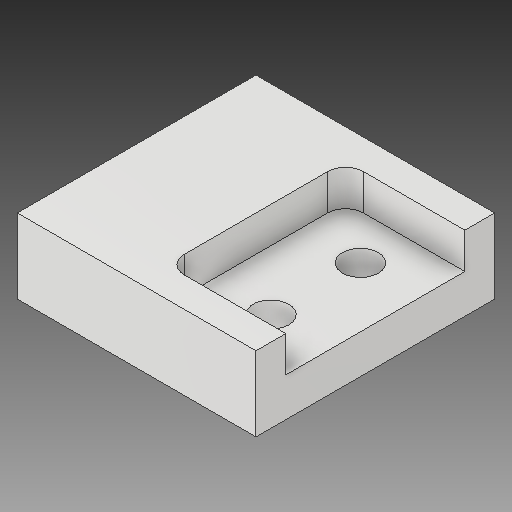
# Autodesk Inventor part: pillar_block
Saved by Autodesk Inventor 2018 (Build 220112000, 112)
## iProperties
Created: 2017-02-15
Part Number: pillar_block
Material: Aluminum 2014-T4
Document SubType Name: Modeling
Designer: steve
Density: 2.8 g/cm^3
Appearance: Satin
Mass: 5.00958 g
Surface Area: 15.2482 cm^2
Volume: 1.78914 cm^3
stock_6_width: 6,250 mm
pillar_block_length: 20,000 mm
pillar_block_width: 20,000 mm
pillar_width: 15,000 mm
stock_3_width: 3,000 mm
pillar_length: 80,000 mm
pillar_plate_length: 60,000 mm
Author: steve
Autodesk Inventor part; units mm, degrees
ref_plane "YZ Plane" through (0, 0, 0) normal (1, 0, 0) x (0, 1, 0)
ref_plane "XZ Plane" through (0, 0, 0) normal (0, 1, 0) x (-1, 0, 0)
ref_plane "XY Plane" through (0, 0, 0) normal (0, 0, 1) x (1, 0, 0)
sketch "Sketch1" plane through (0, 0, 0) normal (0, 1, 0) x (-1, 0, 0)
  line L0 (-10, -10) -> (10, -10)
  line L1 (10, -10) -> (10, 10)
  line L2 (10, 10) -> (-10, 10)
  line L3 (-10, 10) -> (-10, -10)
  line L4 (-10, -10) -> (10, 10) construction
  line L5 (10, -10) -> (-10, 10) construction
  point P0 (0, 0)
  dimension "d0" = 20
  dimension "d1" = 20
  constraints: 12 end point, 2 midpoint, 2 parallel, 1 horizontal, 1 perpendicular
  measures "d0" distance of L0.end L1.end
  measures "d1" distance of L0.start L0.end
extrude "Extrusion1" add sketch "Sketch1" along normal blind 6.25
sketch "Sketch2" plane through (0, 6.25, 0) normal (0, 1, 0) x (1, 0, 0)
  line L0 (10, -7.5) -> (0, -7.5)
  line L1 (0, -7.5) -> (0, 7.5)
  line L2 (0, 7.5) -> (10, 7.5)
  line L3 (10, 7.5) -> (10, -7.5)
  line L4 (10, -10) -> (10, 10) projected
  line L5 (0, 0) -> (15, 0) construction
  line L6 (-15, 0) -> (20, 0) construction
  line L7 (-10, 10) -> (-10, -10) construction
  point P0 (0, 0)
  dimension "d4" = 15
  dimension "d5" = 10
  constraints: 10 end point, 2 collinear, 2 parallel, 1 horizontal, 1 midpoint, 1 perpendicular
  measures "d4" distance of L0.end L1.end
  measures "d5" distance between parallel lines of L7 L1
extrude "Extrusion2" cut sketch "Sketch2" against normal blind 3
sketch "Sketch3" plane through (0, 3.25, 0) normal (0, 1, 0) x (1, 0, 0)
  line L0 (-14, 0) -> (14, 0) construction
  line L1 (10, -7.5) -> (0, -7.5) construction
  line L2 (10, -7.5) -> (0, -7.5) construction
  line L3 (5, -7.5) -> (5, 18.284) construction
  point P0 (0, 0)
  point P1 (5, -3.75)
  point P2 (5, 3.75)
  dimension "d8" = 7.5
  dimension "d26" = 3.75
  constraints: 2 end point, 2 point on line, 1 midpoint, 1 vertical
  measures "d8" distance of point (5, 3.75) point (5, -3.75)
  measures "d26" distance from line of L0 point (5, 3.75)
hole "Hole1" at (5, 3.25, 3.75) at (5, 3.25, -3.75) direction (0, -1, 0) diameter 3 end through all
sketch "Sketch4" plane through (-10, 0, -10) normal (-1, 0, 0) x (0, 0, 1)
  line L0 (0, 0) -> (20, 0) construction
  line L1 (20, 0) -> (20, 6.25) construction
  line L2 (0, 6.25) -> (20, 6.25) construction
  line L3 (0, 0) -> (0, 6.25) construction
  line L4 (20, 3.125) -> (0, 3.125) construction
  line L5 (10, 0) -> (10, 6.25) construction
  point P0 (16, 3.125)
  point P1 (4, 3.125)
  dimension "d17" = 6
  dimension "d18" = 6
  constraints: 4 end point, 3 midpoint, 2 point on line
  measures "d17" distance from line of L5 point (16, 3.125)
  measures "d18" distance from line of point (4, 3.125) L5
hole "Hole2" at (-10, 3.125, 6) at (-10, 3.125, -6) direction (1, 0, 0) diameter 2.459 depth 8.8 tip angle 118 thread size "M3x0.5" class "6H" standard "ANSI Metric M Profile"
fillet "Fillet1" radius 1.5 2 edges at (0, 4.75, -7.5) (0, 4.75, 7.5)
equation "\"d0\" = pillar_block_width"
equation "\"d1\" = pillar_block_length"
equation "\"d2\" = stock_6_width"
equation "\"d4\" = pillar_width"
equation "\"d6\" = stock_3_width"
equation "\"stock_6_width\" = 6.25"
equation "\"pillar_block_length\" = 20"
equation "\"pillar_block_width\" = 20"
equation "\"pillar_width\" = 15"
equation "\"stock_3_width\" = 3"
equation "\"pillar_length\" = 80"
body "Solid1"
